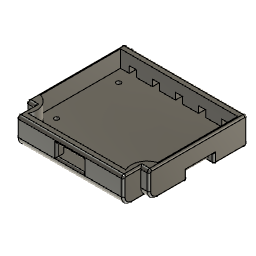
Carcasa Muñeca v5.5 (Autodesk Fusion 360 design; units mm, degrees)
Autodesk Fusion 360 part; units mm, degrees
sketch "Sketch10" plane through (0, 0, 0) normal (0, 0, 1) x (1, 0, 0)
  line L0 (0, -50) -> (0, 50) construction
  line L1 (0, 50) -> (-57, 50)
  line L2 (-57, 50) -> (-57, 0)
  line L3 (0, -50) -> (-45, -50)
  line L4 (-45, -50) -> (-45, -30)
  arc A0 (-57, 0) -> (-45, -30) centre (-7.0663, 2.5735) ccw
  line L5 (0, -50) -> (45, -50)
  line L6 (45, -50) -> (45, -30)
  arc A1 (45, -30) -> (57, 0) centre (7.0663, 2.5735) ccw
  line L7 (57, 50) -> (57, 0)
  line L8 (0, 50) -> (57, 50)
  dimension "d19" = 100
  dimension "d20" = 57
  dimension "d21" = 50
  dimension "d22" = 45
  dimension "d23" = 20
  dimension "d24" = 50
  dimension "d25" = 30
  constraint vertical L0
  constraint midpoint L0 origin
  constraint perpendicular L0 L1
  constraint perpendicular L1 L2
  constraint perpendicular L0 L3
  constraint perpendicular L3 L4
  constraint symmetric L3.start L0 L5.start
  constraint symmetric L1.start L0 L8.start
  constraint symmetric L0 L1.end L7.start
  constraint symmetric L0 L2.end A1.end
  constraint symmetric L0 L3.end L5.end
  constraint symmetric L0 L4.end L6.end
  constraint symmetric L0 A0 A1
  measures "d19" distance of L0.start L0.end
  measures "d20" distance of L0.end L1.end
  measures "d21" distance of L1.end L2.end
  measures "d22" distance of L0.start L3.end
  measures "d23" distance of L3.end L4.end
  measures "d24" radius of A0
  measures "d25" vertical distance of L2.end L4.end
sketch "Sketch12" plane through (0, 0, 0) normal (1, 0, 0) x (0, 1, 0)
  line L0 (0, 15.5) -> (0, -15.5) construction
  line L1 (0, 15.5) -> (60, 15.5)
  line L2 (63, 12.5) -> (63, -12.5)
  arc A0 (63, 12.5) -> (60, 15.5) centre (60, 12.5) ccw
  line L3 (0, 15.5) -> (-65, 15.5)
  line L4 (-68, 12.5) -> (-68, -5.5)
  arc A1 (-65, 15.5) -> (-68, 12.5) centre (-65, 12.5) ccw
  arc A2 (-68, -5.5) -> (-58, -15.5) centre (-58, -5.5) ccw
  arc A3 (60, -15.5) -> (63, -12.5) centre (60, -12.5) ccw
  line L5 (-58, -15.5) -> (60, -15.5)
  dimension "d30" = 3
  dimension "d34" = 3
  dimension "d35" = 10
  dimension "d36" = 18
  dimension "d38" = 3
  dimension "d40" = 25
  dimension "d308" = 65
  dimension "d309" = 60
  constraint vertical L0
  constraint midpoint L0 origin
  constraint perpendicular L0 L1
  constraint perpendicular L1 L2
  constraint tangent L1 A0
  constraint tangent L2 A0
  constraint perpendicular L0 L3
  constraint perpendicular L3 L4
  constraint tangent L4 A1
  constraint tangent L3 A1
  constraint tangent L4 A2
  constraint tangent L2 A3
  constraint tangent A3 L5
  measures "d30" radius of A0
  measures "d34" radius of A1
  measures "d35" radius of A2
  measures "d36" distance of L4.start L4.end
  measures "d38" radius of A3
  measures "d40" distance of L2.start L2.end
  measures "d308" distance of L0.start L3.end
  measures "d309" distance of L0.start L1.end
extrude "Extrude1" add sketch "Sketch12" along normal mid plane 120
ref_plane "PlanoDeObra18" through (-69, -2.5, 0) normal (-1, 0, 0) x (0, -1, 0)
sketch "Boceto31" plane through (-60, 0, 0) normal (-1, 0, 0) x (0, -1, 0)
  line L0 (65, 15.5) -> (-60, 15.5)
  line L1 (-63, 12.5) -> (-63, -12.5)
  arc A0 (-63, -12.5) -> (-60, -15.5) centre (-60, -12.5) ccw
  arc A1 (58, -15.5) -> (68, -5.5) centre (58, -5.5) ccw
  line L2 (68, -5.5) -> (68, 12.5)
  arc A2 (68, 12.5) -> (65, 15.5) centre (65, 12.5) ccw
  arc A3 (-63, -12.5) -> (-60, -15.5) centre (-60, -12.5) ccw
  line L3 (-60, -12.5) -> (-63, -12.5) construction
  line L4 (-60, -12.5) -> (-60, -15.5) construction
  line L5 (-60, -15.5) -> (38, -15.5)
  line L6 (-60, 15.5) -> (45, 15.5)
  line L7 (-63, 12.5) -> (-63, -12.5)
  arc A4 (48, 12.5) -> (44.9876, 15.5) centre (45, 12.5) ccw
  line L8 (45, 12.5) -> (48, 12.5) construction
  line L9 (45, 12.5) -> (44.9876, 15.5) construction
  arc A5 (38, -15.5) -> (48, -5.5) centre (38, -5.5) ccw
  line L10 (38, -5.5) -> (38, -15.5) construction
  line L11 (38, -5.5) -> (48, -5.5) construction
  line L12 (48, -5.5) -> (48, 12.5)
  line L13 (-60, -15.5) -> (58, -15.5)
  arc A6 (-60, 15.5) -> (-63, 12.4998) centre (-60, 12.5) ccw
  line L14 (-60, 12.5) -> (-60, 15.5) construction
  line L15 (-60, 12.5) -> (-63, 12.4998) construction
  dimension "d172" = 3
  dimension "d176" = 3
  dimension "d178" = 10
  dimension "d313" = 98
  dimension "d315" = 105
  dimension "d316" = 3
  constraint coincident A0.centre A3.centre
  constraint coincident A0.end A3.end
  constraint perpendicular L4 L5
  constraint parallel L0 L6
  constraint tangent A3 L7
  constraint tangent L6 A4
  constraint tangent L5 A5
  constraint tangent A5 L12
  constraint tangent A4 L12
  constraint perpendicular L6 L12
  constraint coincident L0.end L6.start
  constraint tangent L6 A6
  constraint tangent L7 A6
  measures "d172" radius of A3
  measures "d176" radius of A4
  measures "d178" radius of A5
  measures "d313" distance of A0.end L5.end
  measures "d315" distance of L0.end L6.end
  measures "d316" radius of A6
extrude "Extruir14" add sketch "Boceto31" along normal blind 9 contours L0 L1 A0 A3 L5 L6 L7 A4 A5 L12 L13 A6
sketch "Boceto32" plane through (60, 0, 0) normal (1, 0, 0) x (0, 1, 0)
  line L0 (60, 15.5) -> (-65, 15.5)
  arc A0 (-65, 15.5) -> (-68, 12.5) centre (-65, 12.5) ccw
  line L1 (-68, 12.5) -> (-68, -5.5)
  arc A1 (-68, -5.5) -> (-58, -15.5) centre (-58, -5.5) ccw
  arc A2 (60, -15.5) -> (63, -12.5) centre (60, -12.5) ccw
  line L2 (63, -12.5) -> (63, 12.5)
  arc A3 (63, 12.5) -> (60, 15.5) centre (60, 12.5) ccw
  arc A4 (63, 12.5) -> (60, 15.5) centre (60, 12.5) ccw
  line L3 (60, 12.5) -> (63, 12.5) construction
  line L4 (60, 12.5) -> (60, 15.5) construction
  line L5 (60, 15.5) -> (-45, 15.5)
  arc A5 (60, -15.5) -> (63, -12.5) centre (60, -12.5) ccw
  line L6 (60, -12.5) -> (60, -15.5) construction
  line L7 (60, -12.5) -> (63, -12.5) construction
  line L8 (-38, -15.5) -> (-38, -5.5) construction
  arc A6 (-48, -5.5) -> (-38, -15.5) centre (-38, -5.5) ccw
  line L9 (-38, -5.5) -> (-48, -5.5) construction
  line L10 (-38, -5.5) -> (-38, -15.5) construction
  arc A7 (-45, 15.5) -> (-48, 12.5004) centre (-45, 12.5) ccw
  line L11 (-45, 12.5) -> (-45, 15.5) construction
  line L12 (-45, 12.5) -> (-48, 12.5004) construction
  line L13 (-48, 12.5004) -> (-48, -5.5)
  line L14 (-38, -15.5) -> (60, -15.5)
  line L15 (-38, -15.5) -> (60, -15.5)
  line L16 (63, 12.5) -> (63, -12.5)
  dimension "d182" = 3
  dimension "d184" = 105
  dimension "d185" = 3
  dimension "d320" = 10
  dimension "d322" = 3
  dimension "d324" = 98
  constraint coincident A3.centre A4.centre
  constraint coincident L0.start A3.end
  constraint perpendicular L4 L5
  constraint coincident A2.centre A5.centre
  constraint coincident A2.start A5.start
  constraint coincident L8.start A6.end
  constraint coincident L8.end A6.centre
  constraint tangent A6 L13
  constraint tangent A2 L14
  constraint perpendicular L6 L15
  constraint tangent A2 L16
  constraint tangent L5 A7
  constraint tangent A6 L14
  constraint tangent A4 L16
  measures "d182" radius of A4
  measures "d184" distance of L0.start L5.end
  measures "d185" radius of A5
  measures "d320" radius of A6
  measures "d322" radius of A7
  measures "d324" distance of L8.start A2.start
extrude "Extruir15" add sketch "Boceto32" along normal blind 9
ref_plane "PlanoDeObra19" through (0, -2.5, -0.5) normal (0, 0, 1) x (0, -1, 0)
sketch "Boceto33" plane through (0, 0, -0.5) normal (0, 0, 1) x (1, 0, 0)
  line L0 (66, 55) -> (-66, 55)
  line L1 (-66, 55) -> (-66, -35)
  line L2 (66, -35) -> (66, 55)
  line L3 (-55, -60) -> (55, -60)
  line L4 (-69, 60) -> (-69, -38)
  line L5 (-60, 60) -> (69, 60)
  line L6 (-60, -65) -> (60, -65)
  arc A0 (-55, -60) -> (-66, -35) centre (-71.233, -52.2225) ccw
  arc A1 (66, -35) -> (55, -60) centre (71.233, -52.2225) ccw
  line L7 (-60, -65) -> (-60, -45)
  line L8 (69, 60) -> (69, -45)
  dimension "d257" = 3
  dimension "d310" = 5
  dimension "d311" = 5
  dimension "d325" = 110
  dimension "d327" = 90
  dimension "d328" = 5
  dimension "d329" = 18
  dimension "d330" = 3
  constraint horizontal L0
  constraint vertical L1
  constraint vertical L2
  constraint horizontal L3
  constraint equal L1 L2
  constraint equal A0 A1
  measures "d257" distance of L1 L4
  measures "d310" distance of L0 L5
  measures "d311" distance of L3 L6
  measures "d325" distance of L3.start L3.end
  measures "d327" distance of L0.end L1.end
  measures "d328" distance of L3.start L7
  measures "d329" radius of A0
  measures "d330" distance of L2 L8
extrude "Extruir16" cut sketch "Boceto33" along normal blind 16 and the other way blind 3
ref_plane "PlanoDeObra20" through (69, 7.5, 15.5) normal (-1, 0, 0) x (0, -1, 0)
sketch "Boceto34" plane through (69, 10, 10) normal (-1, 0, 0) x (0, 0, -1)
  line L0 (25.5, 15) -> (15.5, 15)
  line L1 (15.5, 15) -> (15.5, -15)
  line L2 (15.5, -15) -> (25.5, -15)
  line L3 (25.5, -15) -> (25.5, 15)
  line L4 (25.5, 48) -> (25.5, -50)
  dimension "d205" = 10
  dimension "d206" = 30
  dimension "d331" = 35
  constraint horizontal L0
  constraint vertical L1
  constraint horizontal L2
  constraint vertical L3
  constraint coincident L2.end L4
  measures "d205" distance of L0.start L0.end
  measures "d206" distance of L0.start L2.end
  measures "d331" distance of L2 L4.end
extrude "Extruir17" cut sketch "Boceto34" along normal blind 15
ref_plane "PlanoDeObra21" through (61.5, -5, -10.5) normal (0, 1, 0) x (0, 0, -1)
sketch "Boceto35" plane through (46.5, -5, -6.0333) normal (0, 1, 0) x (1, 0, 0)
  circle A0 centre (15, 4.4667) radius 1.5
  line L0 (22.5, -0.5333) -> (7.5, -0.5333)
  line L1 (7.5, 9.4667) -> (7.5, -0.5333)
  line L2 (7.5, 9.4667) -> (22.5, 9.4667)
  line L3 (22.5, 9.4667) -> (22.5, -0.5333)
  dimension "d210" = 3
  dimension "d290" = 5
  dimension "d291" = 7.5
  dimension "d332" = 5
  dimension "d333" = 7.5
  measures "d210" diameter of A0
  measures "d290" distance of A0.centre L0
  measures "d291" distance of A0.centre L1
  measures "d332" distance of A0.centre L2
  measures "d333" distance of A0.centre L3
extrude "Extruir18" add sketch "Boceto35" along normal up to surface (30 mm away) contours A0
sketch "Boceto43" plane through (-69, 0, 0) normal (-1, 0, 0) x (0, -1, 0)
  line L0 (48, -5.5) -> (48, 12.5)
  arc A0 (48, 12.5) -> (45, 15.5) centre (45, 12.5) ccw
  line L1 (45, 15.5) -> (-60, 15.5)
  arc A1 (-60, 15.5) -> (-63, 12.4998) centre (-60, 12.5) ccw
  line L2 (-63, 12.4998) -> (-63, -12.5)
  arc A2 (-63, -12.5) -> (-60, -15.5) centre (-60, -12.5) ccw
  line L3 (-60, -15.5) -> (38, -15.5)
  arc A3 (38, -15.5) -> (48, -5.5) centre (38, -5.5) ccw
  line L4 (-27, -15.5) -> (3, -15.5)
  line L5 (3, -15.5) -> (3, -5.5)
  line L6 (3, -5.5) -> (-27, -5.5)
  line L7 (-27, -5.5) -> (-27, -15.5)
  dimension "d360" = 30
  dimension "d361" = 10
  dimension "d362" = 35
  constraint horizontal L4
  constraint vertical L5
  constraint horizontal L6
  constraint vertical L7
  constraint coincident L3 L4.start
  measures "d360" distance of L4.start L4.end
  measures "d361" distance of L4.start L6.end
  measures "d362" distance of L3.end L4.end
extrude "Extruir26" cut sketch "Boceto43" against normal blind 15 contours L3 L4 L5 L6 L7
sketch "Boceto44" plane through (0, -3, 0) normal (0, 1, 0) x (-1, 0, 0)
  line L0 (69, -15.5) -> (69, -5.5)
  line L1 (69, -5.5) -> (54, -5.5)
  line L2 (54, -5.5) -> (54, -15.5)
  line L3 (54, -15.5) -> (69, -15.5)
  circle A0 centre (61.5, -10.5) radius 1.5
  dimension "d365" = 3
  dimension "d366" = 7.5
  dimension "d367" = 7.5
  dimension "d368" = 5
  dimension "d369" = 5
  measures "d365" diameter of A0
  measures "d366" distance of L2 A0.centre
  measures "d367" distance of L0 A0.centre
  measures "d368" distance of L1 A0.centre
  measures "d369" distance of L3 A0.centre
extrude "Extruir27" add sketch "Boceto44" along normal up to surface (30 mm away) contours A0
ref_plane "PlanoDeObra22" through (-69, 7.5, 0) normal (-1, 0, 0) x (0, -1, 0)
ref_plane "PlanoDeObra23" through (0, 63, 0) normal (0, 1, 0) x (0, 0, 1)
ref_plane "PlanoDeObra25" through (0, -68, 3.5) normal (0, -1, 0) x (0, 0, -1)
sketch "Boceto36" plane through (0, -68, 3.5) normal (0, -1, 0) x (1, 0, 0)
  line L0 (-14.9998, 6) -> (15.0002, 6)
  line L1 (15.0002, 6) -> (15.0002, -7)
  line L2 (15.0002, -7) -> (-14.9998, -7)
  line L3 (-14.9998, -7) -> (-14.9998, 6)
  line L4 (-14.9998, 6) -> (15.0002, -7) construction
  line L5 (15.0002, 6) -> (-14.9998, -7) construction
  line L6 (-60, -9) -> (60, -9)
  line L7 (-60, 9) -> (60, 9)
  point P0 (0.0002, -0.5)
  dimension "d217" = 30
  dimension "d218" = 13
  dimension "d335" = 3
  constraint horizontal L0
  constraint perpendicular L0 L1
  constraint parallel L0 L2
  constraint parallel L1 L3
  constraint coincident L4 P0
  constraint coincident L5 P0
  measures "d217" distance of L1.end L2.end
  measures "d218" distance of L0.end L1.end
  measures "d335" distance of L0 L7
extrude "Extruir19" cut sketch "Boceto36" against normal blind 8.2397
fillet "Empalme13" radius 2 9 edges at (-69, 63, -0.0001) (-69, 62.1213, -14.6213) (-69, -20.5, -15.5) (-69, 43.5, -15.5) (-69, -45.0711, -12.5711) (-69, -48, 3.5) (-69, -47.1213, 14.6213) (-69, 7.5, 15.5) (-69, 62.1214, 14.6212)
fillet "Empalme14" radius 2 5 edges at (-60, -48, -15.5) (-60, -65.0711, -12.5711) (-60, -68, 3.5) (-60, -67.1213, 14.6213) (-60, -55, 15.5)
fillet "Empalme15" radius 2 9 edges at (69, 42.5, -15.5) (69, 62.1213, -14.6213) (69, 63, 0) (69, 62.1213, 14.6213) (69, 7.5, 15.5) (69, -47.1212, 14.6215) (69, -48, 3.5002) (69, -45.0711, -12.5711) (69, -21.5, -15.5)
fillet "Empalme16" radius 2 5 edges at (60, -55, 15.5) (60, -67.1213, 14.6213) (60, -68, 3.5) (60, -65.0711, -12.5711) (60, -48, -15.5)
sketch "Boceto39" plane through (0, 63, 0) normal (0, 1, 0) x (1, 0, 0)
  line L0 (56, 3.5) -> (48, 3.5)
  line L1 (48, 3.5) -> (48, -4)
  line L2 (48, -4) -> (56, -4)
  line L3 (56, -4) -> (56, 3.5)
  line L4 (67, 12.5) -> (67, -12.5)
  line L5 (30, 3.5) -> (22, 3.5)
  line L6 (22, 3.5) -> (22, -4)
  line L7 (22, -4) -> (30, -4)
  line L8 (30, -4) -> (30, 3.5)
  line L9 (4, 3.5) -> (-4, 3.5)
  line L10 (-4, 3.5) -> (-4, -4)
  line L11 (-4, -4) -> (4, -4)
  line L12 (4, -4) -> (4, 3.5)
  line L13 (-22, 3.5) -> (-30, 3.5)
  line L14 (-30, 3.5) -> (-30, -4)
  line L15 (-30, -4) -> (-22, -4)
  line L16 (-22, -4) -> (-22, 3.5)
  line L17 (-48, 3.5) -> (-56, 3.5)
  line L18 (-56, 3.5) -> (-56, -4)
  line L19 (-56, -4) -> (-48, -4)
  line L20 (-48, -4) -> (-48, 3.5)
  line L21 (-60, -12.5) -> (67, -12.5)
  line L22 (-67, -12.4998) -> (-67, 12.5)
  line L23 (67, 3.6424) -> (-67, 3.6424)
  dimension "d236" = 8
  dimension "d237" = 7.5
  dimension "d239" = 8
  dimension "d240" = 7.5
  dimension "d242" = 8
  dimension "d243" = 7.5
  dimension "d245" = 8
  dimension "d246" = 7.5
  dimension "d248" = 8
  dimension "d249" = 7.5
  dimension "d280" = 18
  dimension "d281" = 18
  dimension "d282" = 18
  dimension "d285" = 18
  dimension "d373" = 11
  dimension "d374" = 11
  constraint horizontal L0
  constraint vertical L1
  constraint horizontal L2
  constraint vertical L3
  constraint horizontal L5
  constraint vertical L6
  constraint horizontal L7
  constraint vertical L8
  constraint horizontal L9
  constraint vertical L10
  constraint horizontal L11
  constraint vertical L12
  constraint horizontal L13
  constraint vertical L14
  constraint horizontal L15
  constraint vertical L16
  constraint horizontal L17
  constraint vertical L18
  constraint horizontal L19
  constraint vertical L20
  constraint coincident L4 L23.start
  constraint coincident L22 L23.end
  constraint perpendicular L22 L23
  measures "d236" distance of L0.start L0.end
  measures "d237" distance of L0.start L2.end
  measures "d239" distance of L5.start L5.end
  measures "d240" distance of L5.start L7.end
  measures "d242" distance of L9.start L9.end
  measures "d243" distance of L9.start L11.end
  measures "d245" distance of L13.start L13.end
  measures "d246" distance of L13.start L15.end
  measures "d248" distance of L17.start L17.end
  measures "d249" distance of L17.start L19.end
  measures "d280" distance of L1 L8
  measures "d281" distance of L6 L12
  measures "d282" distance of L10 L16
  measures "d285" distance of L14 L20
  measures "d373" distance of L3 L4
  measures "d374" distance of L17.end L22
extrude "Extruir22" cut sketch "Boceto39" against normal blind 8
sketch "Boceto40" plane through (0, 0, -3.5) normal (0, 0, 1) x (-1, 0, 0)
  line L0 (66, -55) -> (66, 35)
  line L1 (-15.0002, 60) -> (-55, 60)
  line L2 (-66, 35) -> (-66, -55)
  line L3 (-66, -55) -> (-56, -55)
  line L4 (14.9998, 60) -> (14.9998, 68)
  line L5 (-15.0002, 68) -> (-15.0002, 60)
  arc A0 (-66, 35) -> (-55, 60) centre (-71.233, 52.2225) ccw
  arc A1 (55, 60) -> (66, 35) centre (71.233, 52.2225) ccw
  line L6 (-56, -55) -> (-56, -63)
  line L7 (-56, -63) -> (-48, -63)
  line L8 (-48, -63) -> (-48, -55)
  line L9 (-48, -55) -> (-30, -55)
  line L10 (-30, -55) -> (-30, -63)
  line L11 (-30, -63) -> (-22, -63)
  line L12 (-22, -63) -> (-22, -55)
  line L13 (-22, -55) -> (-4, -55)
  line L14 (-4, -55) -> (-4, -63)
  line L15 (-4, -63) -> (4, -63)
  line L16 (4, -63) -> (4, -55)
  line L17 (4, -55) -> (22, -55)
  line L18 (22, -55) -> (22, -63)
  line L19 (22, -63) -> (30, -63)
  line L20 (30, -63) -> (30, -55)
  line L21 (30, -55) -> (48, -55)
  line L22 (48, -55) -> (48, -63)
  line L23 (48, -63) -> (56, -63)
  line L24 (56, -63) -> (56, -55)
  line L25 (56, -55) -> (66, -55)
  line L26 (55, 60) -> (14.9998, 60)
  line L27 (14.9998, 68) -> (-15.0002, 68)
sketch "Boceto41" plane through (0, 0, -3.5) normal (0, 0, 1) x (1, 0, 0)
  circle A0 centre (-53, 40) radius 2.5
  circle A1 centre (-53, -30) radius 2.5
  circle A2 centre (53, 40) radius 2.5
  circle A3 centre (53, -30) radius 2.5
  line L0 (53, -30) -> (-53, -30)
  line L1 (-53, -30) -> (-53, 40)
  line L2 (-53, 40) -> (53, 40)
  line L3 (53, 40) -> (53, -30)
  line L4 (-66, -35) -> (-66, 55)
  line L5 (66, 55) -> (66, -35)
  line L6 (-66, 55) -> (66, 55)
  line L7 (55, -60) -> (15.0002, -60)
  line L8 (-14.9998, -60) -> (-55, -60)
  dimension "d260" = 5
  dimension "d261" = 5
  dimension "d262" = 5
  dimension "d264" = 106
  dimension "d265" = 70
  dimension "d266" = 5
  dimension "d267" = 106
  dimension "d268" = 70
  dimension "d375" = 13
  dimension "d376" = 13
  dimension "d377" = 15
  dimension "d378" = 30
  constraint coincident A3.centre L0.start
  constraint coincident A1.centre L0.end
  constraint horizontal L0
  constraint coincident A0.centre L1.end
  constraint perpendicular L0 L1
  constraint coincident A2.centre L2.end
  measures "d260" diameter of A0
  measures "d261" diameter of A1
  measures "d262" diameter of A2
  measures "d264" distance of A0.centre A2.centre
  measures "d265" distance of A0.centre A1.centre
  measures "d266" diameter of A3
  measures "d267" distance of A1.centre A3.centre
  measures "d268" distance of A2.centre A3.centre
  measures "d375" distance of A0.centre L4
  measures "d376" distance of L3 L5
  measures "d377" distance of L2 L6
  measures "d378" distance of L0 L7
extrude "Extruir23" cut sketch "Boceto41" against normal blind 12 contours A0 L1 L2 | A0 L1 L2 | A2 L2 L3 | A2 L2 L3 | A1 L0 L1 | A1 L0 L1 | A3 L0 L3 | A3 L0 L3
fillet "Empalme19" radius 2 8 edges at (54, 10, -15.5) (60.5, -5, -15.5) (68.4142, -5, -14.9142) (69, -5, -9.5) (69, 25, -9.5) (68.4142, 25, -14.9142) (60.5, 25, -15.5) (69, 10, -5.5)
fillet "Empalme20" radius 2 8 edges at (-69, 12, -5.5) (-69, -3, -9.5) (-68.4142, -3, -14.9142) (-60.5, -3, -15.5) (-60.5, 27, -15.5) (-68.4142, 27, -14.9142) (-69, 27, -9.5) (-54, 12, -15.5)
fillet "Empalme21" radius 2 4 edges at (0.0002, -68, -3.5) (-14.9998, -68, 3) (0.0002, -68, 9.5) (15.0002, -68, 3)
sketch "Boceto45" plane through (0, 0, -15.5) normal (0, 0, -1) x (1, 0, 0)
  line L0 (-52, -29) -> (-67, -29)
  line L1 (-67, -29) -> (-67, -60)
  line L2 (-67, -60) -> (67, -60)
  line L3 (67, -60) -> (67, -27)
  line L4 (67, -27) -> (52, -27)
  line L5 (52, -27) -> (52, 7)
  line L6 (52, 7) -> (67, 7)
  line L7 (67, 7) -> (67, 38)
  line L8 (67, 38) -> (58, 38)
  line L9 (58, 38) -> (58, 58)
  line L10 (58, 58) -> (-58, 58)
  line L11 (-58, 58) -> (-58, 38)
  line L12 (-58, 38) -> (-67, 38)
  line L13 (-67, 38) -> (-67, 5)
  line L14 (-67, 5) -> (-52, 5)
  line L15 (-52, 5) -> (-52, -29)
  circle A0 centre (-53, 30) radius 2.5
  circle A1 centre (53, -40) radius 2.5
  circle A2 centre (-53, -40) radius 2.5
  circle A3 centre (53, 30) radius 2.5
  circle A4 centre (53, -40) radius 3.5
  circle A5 centre (53, 30) radius 3.5
  circle A6 centre (-53, -40) radius 3.5
  circle A7 centre (-53, 30) radius 3.5
  dimension "d385" = 7
  dimension "d386" = 7
  dimension "d387" = 7
  dimension "d388" = 7
  constraint concentric A1 A4
  constraint concentric A3 A5
  constraint concentric A2 A6
  constraint concentric A0 A7
  measures "d385" diameter of A4
  measures "d386" diameter of A5
  measures "d387" diameter of A6
  measures "d388" diameter of A7
extrude "Extruir29" cut sketch "Boceto45" against normal blind 2.5 contours A4 | A5 | A6 | A7
fillet "Empalme22" radius 1 4 edges at (49.7369, 38.7343, -15.5) (49.7369, -31.2657, -15.5) (-56.2631, 38.7343, -15.5) (-56.2631, -31.2657, -15.5)
